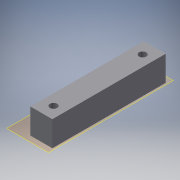
# Autodesk Inventor part: tg
Saved by Autodesk Inventor 2017 (Build 210142000, 142)
## iProperties
Part Number: tg
Material: Générique
Document SubType Name: Modeling
Designer: Thomas
Density: 1 g/cm^3
Appearance: Par défaut
Author: Thomas
Autodesk Inventor part; units mm, degrees
note: some values were not read from the file. Chosen so that the rebuilt part matches the saved one: sketch regions of "Extrusion1".
ref_plane "YZ Plane" through (0, 0, 0) normal (1, 0, 0) x (0, 1, 0)
ref_plane "XZ Plane" through (0, 0, 0) normal (0, 1, 0) x (-1, 0, 0)
ref_plane "XY Plane" through (0, 0, 0) normal (0, 0, 1) x (1, 0, 0)
ref_plane "Plan de construction1" through (0, 0, 0) normal (0, 0, 1) x (1, 0, 0)
sketch "Esquisse1" plane through (0, 0, 0) normal (0, 0, 1) x (1, 0, 0)
  circle A0 centre (36.4553, 35.5016) radius 2.25 projected
  line L0 (29.7194, 25.7651) -> (43.1911, 25.7651) projected
  line L1 (43.1911, 25.7651) -> (43.1911, 43.0016) projected
  line L2 (43.1911, 43.0016) -> (29.7194, 43.0016) projected
  line L3 (29.7194, 43.0016) -> (29.7194, 25.7651) projected
  circle A1 centre (36.4553, -19.4032) radius 2.25 projected
  circle A2 centre (36.4553, 35.5016) radius 2.25 projected
  circle A3 centre (25.0518, -6.7548) radius 2.15 projected
  circle A4 centre (25.0518, 23.2452) radius 2.15 projected
  line L4 (43.1911, 43.0016) -> (43.1911, -26.9032) projected
  line L5 (29.7194, 43.0016) -> (43.1911, 43.0016) projected
  line L6 (29.7194, 28.2452) -> (29.7194, 43.0016) projected
  line L7 (29.7194, 28.2452) -> (19.7194, 28.2452) projected
  line L8 (19.7194, 28.2452) -> (19.7194, 19.2452) projected
  line L9 (19.7194, 19.2452) -> (38.63, 19.2452) projected
  line L10 (38.63, 19.2452) -> (38.63, -2.9032) projected
  line L11 (38.63, -2.9032) -> (19.7194, -2.9032) projected
  line L12 (19.7194, -2.9032) -> (19.7194, -11.9032) projected
  line L13 (19.7194, -11.9032) -> (29.7194, -11.9032) projected
  line L14 (29.7194, -26.9032) -> (29.7194, -11.9032) projected
  line L15 (43.1911, -26.9032) -> (29.7194, -26.9032) projected
  line L16 (43.1911, 43.0016) -> (29.7194, 43.0016)
  line L17 (29.7194, 43.0016) -> (29.7194, -26.9032)
  line L18 (29.7194, -26.9032) -> (43.1911, -26.9032)
  line L19 (43.1911, -26.9032) -> (43.1911, 43.0016)
  point P0 (0, 0)
  constraints: 8 end point, 2 parallel, 1 horizontal, 1 perpendicular
extrude "Extrusion1" add sketch "Esquisse1" along normal blind 15.5 contours L3 L2 L1 L0 | L0 L4 L15 L14 L17 L11 L10 L9 | L9 L10 L11 L17
